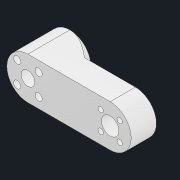
# Autodesk Inventor part: scara-base17
Saved by Autodesk Inventor 2022 (Build 260153000, 153)
## iProperties
Created: 2021-10-12
Part Number: scara-base17
Material: ABS プラスチック
Document SubType Name: Modeling
Designer: Yuta Kage
Density: 1.06 g/cm^3
Appearance: 滑らか - 白
Mass: 32.092 g
Surface Area: 93.3551 cm^2
Volume: 30.2755 cm^3
Description: 印刷
Author: Yuta Kage
Autodesk Inventor part; units mm, degrees
ref_plane "YZ Plane" through (0, 0, 0) normal (1, 0, 0) x (0, 1, 0)
ref_plane "XZ Plane" through (0, 0, 0) normal (0, 1, 0) x (-1, 0, 0)
ref_plane "XY Plane" through (0, 0, 0) normal (0, 0, 1) x (1, 0, 0)
sketch "スケッチ1" plane through (0, 0, 0) normal (0, 0, 1) x (1, 0, 0)
  line L0 (-24.5, 0) -> (24.5, 0) construction
  line L1 (-24.5, -12.5) -> (24.5, -12.5)
  line L2 (24.5, 12.5) -> (-24.5, 12.5)
  arc A0 (-24.5, 12.5) -> (-24.5, -12.5) centre (-24.5, 0) ccw
  arc A1 (24.5, -12.5) -> (24.5, 12.5) centre (24.5, 0) ccw
  point P0 (0, 0)
  dimension "d0" = 49
  dimension "d1" = 12.5
  constraints: 8 end point, 4 point on circle, 4 tangent, 2 centre point, 1 horizontal, 1 midpoint, 1 parallel
  measures "d0" distance of L0.start L0.end
  measures "d1" radius of A1
extrude "押し出し1" add sketch "スケッチ1" along normal mid plane 15
sketch "スケッチ2" plane through (0, 0, 7.5) normal (0, 0, 1) x (1, 0, 0)
  arc A0 (24.5, -12.5) -> (24.5, 12.5) centre (24.5, 0) ccw projected
  circle A1 centre (24.5, 0) radius 5.2
  point P0 (0, 0)
  dimension "d4" = 10.4
  constraints: 1 centre point, 1 coincident
  measures "d4" diameter of A1
extrude "押し出し2" cut sketch "スケッチ2" against normal blind 50
sketch "スケッチ3" plane through (0, 0, 7.5) normal (0, 0, 1) x (1, 0, 0)
  circle A0 centre (24.5, 0) radius 5.2 projected
  circle A1 centre (24.5, 0) radius 8
  point P0 (0, 0)
  point P1 (30.1569, 5.6569)
  point P2 (18.8431, 5.6569)
  point P3 (18.8431, -5.6569)
  point P4 (30.1569, -5.6569)
  dimension "d7" = 16
  dimension "d10" = 360
  dimension "d40" = 5.6569
  constraints: 1 coincident, 8 other
  measures "d40" horizontal distance of A0.centre point (18.843, 5.657)
hole "穴1" at (30.1569, 5.6569, 7.5) at (18.8431, 5.6569, 7.5) at (18.8431, -5.6569, 7.5) at (30.1569, -5.6569, 7.5) direction (0, 0, -1) diameter 3.2 end through all clearance for "Socket Head Cap Screw" size "M3" standard "Ansi Metric M Profile"
sketch "スケッチ8" plane through (0, 0, -7.5) normal (0, 0, -1) x (-1, 0, 0)
  circle A0 centre (-18.8431, -5.6569) radius 1.6 projected
  circle A1 centre (-30.1569, 5.6569) radius 1.6 projected
  circle A2 centre (-18.8431, 5.6569) radius 1.6 projected
  circle A3 centre (-30.1569, -5.6569) radius 1.6 projected
  circle A4 centre (-24.5, 0) radius 5.2 projected
  arc A5 (-24.5, 12.5) -> (-24.5, -12.5) centre (-24.5, 0) ccw projected
  line L0 (-24.5, -12.5) -> (24.5, -12.5) projected
  arc A6 (24.5, -12.5) -> (24.5, 12.5) centre (24.5, 0) ccw projected
  line L1 (24.5, 12.5) -> (-24.5, 12.5) projected
  line L2 (-24.5, -12.5) -> (24.5, -12.5) projected
  circle A7 centre (24.5, 0) radius 12.5
  point P0 (0, 0)
  point P1 (24.5, 12.5)
  constraints: 1 coincident, 3 other
extrude "押し出し6" add sketch "スケッチ8" along normal blind 10 contours A6 A7
sketch "スケッチ4" plane through (0, 0, 7.5) normal (0, 0, 1) x (1, 0, 0)
  arc A0 (-24.5, 12.5) -> (-24.5, -12.5) centre (-24.5, 0) ccw projected
  circle A1 centre (-24.5, 0) radius 9
  point P0 (0, 0)
  point P1 (-18.136, -6.364)
  point P2 (-18.136, 6.364)
  point P3 (-30.864, 6.364)
  point P4 (-30.864, -6.364)
  dimension "d19" = 18
  dimension "d22" = 360
  dimension "d42" = 0
  constraints: 1 coincident, 8 other
  measures "d42" vertical distance of point (-30.864, 6.364) point (-18.136, 6.364)
hole "穴2" at (-18.136, -6.364, 7.5) at (-18.136, 6.364, 7.5) at (-30.864, 6.364, 7.5) at (-30.864, -6.364, 7.5) direction (0, 0, -1) diameter 4.3 end through all clearance for "Socket Head Cap Screw" size "M4" standard "Ansi Metric M Profile"
sketch "スケッチ5" plane through (0, 0, 7.5) normal (0, 0, 1) x (1, 0, 0)
  arc A0 (-24.5, 12.5) -> (-24.5, -12.5) centre (-24.5, 0) ccw projected
  circle A1 centre (-24.5, 0) radius 4.1
  point P0 (0, 0)
  dimension "d31" = 8.2
  constraints: 1 centre point, 1 coincident
  measures "d31" diameter of A1
extrude "押し出し3" cut sketch "スケッチ5" against normal blind 50
chamfer "面取り1" distance 10 angle 45 1 edges at (-12, 0, -7.5)
